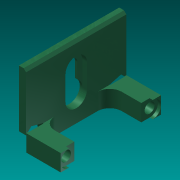
# Autodesk Inventor part: MotorClipV4
Saved by Autodesk Inventor 2013 (Build 170138000, 138)
## iProperties
Created: 2013-08-18
Part Number: MotorClipV4
Material: ABS Plastic
Document SubType Name: Modeling
Designer: Sawaiz
Density: 1 g/cm^3
Author: Sawaiz
Autodesk Inventor part; units mm, degrees
ref_plane "YZ Plane" through (0, 0, 0) normal (1, 0, 0) x (0, 1, 0)
ref_plane "XZ Plane" through (0, 0, 0) normal (0, 1, 0) x (-1, 0, 0)
ref_plane "XY Plane" through (0, 0, 0) normal (0, 0, 1) x (1, 0, 0)
sketch "Sketch1" plane through (0, 0, 0) normal (0, 0, 1) x (1, 0, 0)
  line L0 (-14, 0) -> (-21, 0)
  line L1 (-21, 0) -> (-21, 7)
  line L2 (-21, 7) -> (-14, 7)
  line L3 (-14, 7) -> (-14, 0)
  line L4 (14, 0) -> (21, 0)
  line L5 (21, 0) -> (21, 7)
  line L6 (21, 7) -> (14, 7)
  line L7 (14, 7) -> (14, 0)
  point P0 (0, 0)
  dimension "d0" = 7
  dimension "d2" = 7
  dimension "d3" = 42
  dimension "d4" = 7
  dimension "d5" = 7
  dimension "d6" = 14
  constraints: 16 end point, 4 parallel, 2 horizontal, 2 perpendicular
  measures "d0" distance of L0.end L1.end
  measures "d2" distance of L4.end L5.end
  measures "d3" distance between parallel lines of L1 L5
  measures "d4" distance of L1.end L2.end
  measures "d5" distance of L5.end L6.end
  measures "d6" distance from line of L7 point (0, 0)
extrude "Extrusion1" add sketch "Sketch1" against normal blind 13.716
sketch "Sketch2" plane through (0, 0, -13.716) normal (0, 0, -1) x (-1, 0, 0)
  line L0 (14, 0) -> (21, 0) projected
  line L1 (21, 0) -> (21, 7) projected
  line L2 (21, 7) -> (14, 7) projected
  line L3 (14, 7) -> (14, 0) projected
  line L4 (21, 0) -> (-21, 0)
  line L5 (-21, 0) -> (-21, 30)
  line L6 (-21, 30) -> (21, 30)
  line L7 (21, 30) -> (21, 0)
  point P0 (0, 0)
  dimension "d9" = 30
  constraints: 8 end point, 2 parallel, 1 horizontal, 1 perpendicular
  measures "d9" distance of L4.end L5.end
extrude "Extrusion2" add sketch "Sketch2" along normal blind 3
chamfer "Chamfer1" distance 1 angle 45 1 edges at (0, 30, -13.716)
sketch "Sketch3" plane through (0, 0, -13.716) normal (0, 0, 1) x (1, 0, 0)
  line L0 (-21, 29) -> (21, 29) projected
  line L1 (14, 0) -> (-14, 0) projected
  line L2 (0, 0) -> (0, 29)
  circle A0 centre (0, 10) radius 4.5
  circle A1 centre (0, 20) radius 2.5
  line L3 (-2.5, 20) -> (-2.5, 6.2583)
  line L4 (2.5, 20) -> (2.5, 6.2583)
  dimension "d16" = 9
  dimension "d18" = 5
  dimension "d19" = 10
  dimension "d20" = 20
  constraints: 6 end point, 4 point on circle, 2 centre point, 2 parallel, 2 point on line, 2 tangent, 1 midpoint
  measures "d16" diameter of A0
  measures "d18" diameter of A1
  measures "d19" distance from line of A0.centre L1
  measures "d20" distance from line of L1 A1.centre
extrude "Extrusion3" cut sketch "Sketch3" against normal through all
sketch "Sketch4" plane through (0, 0, -13.716) normal (0, 0, 1) x (1, 0, 0)
  arc A0 (-2.5, 13.7417) -> (2.5, 13.7417) centre (0, 10) ccw projected
  line L0 (-2.5, 13.7417) -> (-2.5, 20) projected
  arc A1 (2.5, 20) -> (-2.5, 20) centre (0, 20) ccw projected
  line L1 (2.5, 20) -> (2.5, 13.7417) projected
  line L2 (21, 29) -> (21, 7) projected
  circle A2 centre (0, 20) radius 4.5
  line L3 (-4.5, 20) -> (-4.5, 10)
  line L4 (4.5, 10) -> (4.5, 20)
  point P0 (0, 0)
  dimension "d23" = 9
  constraints: 4 end point, 4 point on circle, 2 parallel, 2 tangent, 1 centre point, 1 coincident
  measures "d23" diameter of A2
extrude "Extrusion4" cut sketch "Sketch4" against normal blind 2
sketch "Sketch5" plane through (0, 0, 0) normal (0, 0, 1) x (1, 0, 0)
  line L0 (-14, 7) -> (-14, 0) projected
  line L1 (-21, 0) -> (-21, 7) projected
  line L2 (14, 0) -> (21, 0) projected
  line L3 (21, 0) -> (21, 7) projected
  line L4 (21, 7) -> (14, 7) projected
  line L5 (14, 7) -> (14, 0) projected
  line L6 (-21, 3.5) -> (-14, 3.5)
  line L7 (14, 3.5) -> (21, 3.5)
  point P0 (0, 0)
  point P1 (-17.5, 3.5)
  point P2 (17.5, 3.5)
  dimension "d26" = 35
  dimension "d28" = 3.5
  dimension "d29" = 3.5
  constraints: 6 midpoint, 4 end point
  measures "d26" distance of point (17.5, 3.5) point (-17.5, 3.5)
  measures "d28" distance of L6.start point (-17.5, 3.5)
  measures "d29" distance from line of L3 point (17.5, 3.5)
hole "Hole1" at (-17.5, 3.5, 0) at (17.5, 3.5, 0) direction (0, 0, -1) diameter 4.2 end through all
fillet "Fillet1" radius 5 2 edges at (-14, 3.5, -13.716) (14, 3.5, -13.716)
sketch "Sketch6" plane through (0, 0, 0) normal (0, 0, 1) x (1, 0, 0)
  circle A0 centre (-17.5, 3.5) radius 2.1 projected
  line L0 (-14, 0) -> (-21, 0) projected
  line L1 (-14, 7) -> (-14, 0) projected
  line L2 (-21, 7) -> (-14, 7) projected
  line L3 (-21, 0) -> (-21, 7) projected
  circle A1 centre (17.5, 3.5) radius 2.1 projected
  line L4 (14, 0) -> (21, 0) projected
  line L5 (21, 0) -> (21, 7) projected
  line L6 (21, 7) -> (14, 7) projected
  line L7 (14, 7) -> (14, 0) projected
  arc A2 (-17.5, 7) -> (-17.5, 0) centre (-17.5, 3.5) ccw
  arc A3 (17.5, 0) -> (17.5, 7) centre (17.5, 3.5) ccw
  line L8 (17.5, 7) -> (21, 7)
  line L9 (21, 7) -> (21, 0)
  line L10 (21, 0) -> (17.5, 0)
  line L11 (-17.5, 0) -> (-21, 0)
  line L12 (-21, 0) -> (-21, 7)
  line L13 (-17.5, 7) -> (-21, 7)
  point P0 (0, 0)
  constraints: 12 end point, 4 midpoint, 4 point on circle, 4 tangent, 2 centre point, 2 coincident, 2 collinear, 2 perpendicular
ref_plane "Work Plane1" through (-21, 0, 0.82) normal (0, 0, -1) x (0, 1, 0)
extrude "Extrusion5" add sketch "Sketch6" along normal up to surface (0.82 mm away) contours L0 L3 A2 | L3 L2 A2 | A3 L5 L4 | A3 L6 L5
sketch "Sketch7" plane through (0, 0, 0) normal (0, 0, 1) x (1, 0, 0)
  arc A0 (-21, 3.5) -> (-17.5, 0) centre (-17.5, 3.5) ccw projected
  line L0 (-14, 0) -> (-17.5, 0) projected
  line L1 (-14, 7) -> (-14, 0) projected
  line L2 (-17.5, 7) -> (-14, 7) projected
  arc A1 (-17.5, 7) -> (-21, 3.5) centre (-17.5, 3.5) ccw projected
  circle A2 centre (-17.5, 3.5) radius 2.1 projected
  circle A3 centre (17.5, 3.5) radius 2.1 projected
  arc A4 (17.5, 0) -> (21, 3.5) centre (17.5, 3.5) ccw projected
  arc A5 (21, 3.5) -> (17.5, 7) centre (17.5, 3.5) ccw projected
  line L3 (17.5, 7) -> (14, 7) projected
  line L4 (14, 7) -> (14, 0) projected
  line L5 (14, 0) -> (17.5, 0) projected
  point P0 (0, 0)
extrude "Extrusion6" cut sketch "Sketch7" against normal blind 0.5
sketch "Sketch8" plane through (0, 0, -16.716) normal (0, 0, -1) x (-1, 0, 0)
  circle A0 centre (17.5, 3.5) radius 2.1 projected
  circle A1 centre (-17.5, 3.5) radius 2.1 projected
  line L0 (-12.64, 2.1615) -> (-13.9108, 7.0396) projected
  line L1 (-16.2292, -1.3782) -> (-12.64, 2.1615) projected
  line L2 (-21.0892, -0.0396) -> (-16.2292, -1.3782) projected
  line L3 (-22.36, 4.8385) -> (-21.0892, -0.0396) projected
  line L4 (-18.7708, 8.3782) -> (-22.36, 4.8385) projected
  line L5 (-13.9108, 7.0396) -> (-18.7708, 8.3782) projected
  circle A2 centre (-17.5, 3.5) radius 1.6532 projected
  line L6 (21.0628, -0.0662) -> (22.3699, 4.8024) projected
  line L7 (16.1929, -1.3686) -> (21.0628, -0.0662) projected
  line L8 (12.6301, 2.1976) -> (16.1929, -1.3686) projected
  line L9 (13.9372, 7.0662) -> (12.6301, 2.1976) projected
  line L10 (18.8071, 8.3686) -> (13.9372, 7.0662) projected
  line L11 (22.3699, 4.8024) -> (18.8071, 8.3686) projected
  circle A3 centre (17.5, 3.5) radius 1.6532 projected
  point P0 (0, 0)
extrude "Extrusion7" cut sketch "Sketch8" against normal blind 3.175 contours L1 L2 L3 L4 L5 L0 | L7 L8 L9 L10 L11 L6
equation "\"d7\" = StretcherDepth"
equation "\"d28\" = d29"
equation "\"StretcherDepth\" = 13.716"
body "Solid1"
